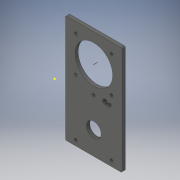
# Autodesk Inventor part: y gearing adapter
Saved by Autodesk Inventor 2019 (Build 230136000, 136)
## iProperties
Created: 2018-07-27
Part Number: y gearing adapter
Material: Generic
Document SubType Name: Modeling
Designer: torba
Density: 1 g/cm^3
Appearance: Gray
Author: torba
Autodesk Inventor part; units mm, degrees
ref_plane "YZ Plane" through (0, 0, 0) normal (1, 0, 0) x (0, 1, 0)
ref_plane "XZ Plane" through (0, 0, 0) normal (0, 1, 0) x (-1, 0, 0)
ref_plane "XY Plane" through (0, 0, 0) normal (0, 0, 1) x (1, 0, 0)
sketch "Sketch1" plane through (0, 0, 0) normal (0, 0, 1) x (1, 0, 0)
  arc A0 (44.2015, -79.5823) -> (38.6015, -79.5823) centre (41.4015, -79.5823) ccw
  arc A1 (38.6015, -85.1823) -> (44.2015, -85.1823) centre (41.4015, -85.1823) ccw
  line L0 (38.6015, -85.1823) -> (38.6015, -79.5823)
  line L1 (44.2015, -79.5823) -> (44.2015, -85.1823)
  arc A2 (39.4335, -50.3778) -> (112.9665, -50.3778) centre (76.2, -50.3778) ccw
  arc A3 (112.9665, -44.7898) -> (39.4335, -44.7898) centre (76.2, -44.7898) ccw
  line L2 (39.4335, -50.3778) -> (39.4335, -44.7898)
  line L3 (112.9665, -44.7898) -> (112.9665, -50.3778)
  line L4 (44.2015, -9.9853) -> (44.2015, -15.5853)
  arc A4 (44.2015, -9.9853) -> (38.6015, -9.9853) centre (41.4015, -9.9853) ccw
  line L5 (38.6015, -15.5853) -> (38.6015, -9.9853)
  arc A5 (38.6015, -15.5853) -> (44.2015, -15.5853) centre (41.4015, -15.5853) ccw
  line L6 (108.1985, -85.1823) -> (108.1985, -79.5823)
  arc A6 (108.1985, -85.1823) -> (113.7985, -85.1823) centre (110.9985, -85.1823) ccw
  line L7 (113.7985, -79.5823) -> (113.7985, -85.1823)
  arc A7 (113.7985, -79.5823) -> (108.1985, -79.5823) centre (110.9985, -79.5823) ccw
  line L8 (108.1985, -15.5853) -> (108.1985, -9.9853)
  arc A8 (113.7985, -9.9853) -> (108.1985, -9.9853) centre (110.9985, -9.9853) ccw
  line L9 (113.7985, -9.9853) -> (113.7985, -15.5853)
  arc A9 (108.1985, -15.5853) -> (113.7985, -15.5853) centre (110.9985, -15.5853) ccw
  circle A10 centre (76.2, -47.5838) radius 1.27
  line L10 (6.35, 0.0014) -> (6.35, -109.7489)
  line L11 (152.4, 0) -> (0, 0)
  line L12 (146.05, 0.0027) -> (146.05, -109.7476)
  line L13 (0, -109.7503) -> (152.4, -109.7503)
  line L14 (21.2, 7.4162) -> (131.2, 7.4162)
  line L15 (131.2, 7.4162) -> (131.2, -102.5838)
  line L16 (131.2, -102.5838) -> (21.2, -102.5838)
  line L17 (21.2, -102.5838) -> (21.2, 7.4162)
  line L18 (21.2, 7.4162) -> (131.2, -102.5838) construction
  line L19 (131.2, 7.4162) -> (21.2, -102.5838) construction
  dimension "d0" = 2.8
  dimension "d1" = 36.7665
  dimension "d2" = 2.54
  dimension "d3" = 90
  dimension "d4" = 90
  dimension "d5" = 90
  dimension "d6" = 90
  dimension "d7" = 109.7503
  dimension "d8" = 32.2515
  dimension "d9" = 33.0835
  dimension "d10" = 101.8485
  dimension "d11" = 139.7
  dimension "d12" = 6.35
  dimension "d13" = 38.6015
  dimension "d14" = 6.35
  dimension "d15" = 0.0027
  dimension "d16" = 37.8515
  dimension "d17" = 109.7476
  dimension "d18" = 9.9853
  dimension "d19" = 69.597
  dimension "d20" = 75.197
  dimension "d21" = 79.5823
  dimension "d22" = 44.7898
  dimension "d23" = 50.3778
  dimension "d24" = 47.5838
  dimension "d25" = 69.85
  dimension "d26" = 9.9853
  dimension "d27" = 79.5823
  dimension "d28" = 0.0014
  dimension "d29" = 109.7489
  dimension "d30" = 146.05
  dimension "d31" = 146.05
  dimension "d32" = 110
  dimension "d33" = 110
  dimension "d34" = 17.4015
  constraints: 40 end point, 24 tangent, 20 point on circle, 11 centre point, 10 parallel, 2 horizontal, 2 midpoint, 1 equal radius, 1 perpendicular, 1 vertical
  measures "d0" radius of A8
  measures "d1" radius of A3
  measures "d2" diameter of A10
  measures "d3" angle of L11 L9
  measures "d4" angle of L11 L8
  measures "d5" angle of L11 L1
  measures "d6" angle of L11 L0
  measures "d7" distance between parallel lines of L11 L13
  measures "d8" distance between parallel lines of L12 L7
  measures "d9" distance between parallel lines of L12 L3
  measures "d10" distance between parallel lines of L12 L4
  measures "d11" distance between parallel lines of L12 L10
  measures "d12" distance from line of L11.start L12
  measures "d13" distance from line of L11.start L9
  measures "d14" distance from line of L13.end L12
  measures "d15" distance from line of L12.start L11
  measures "d16" distance from line of L12.start L8
  measures "d17" distance from line of L12.end L11
  measures "d18" distance from line of L9.start L11
  measures "d19" distance from line of L9.start L1
  measures "d20" distance from line of L9.start L0
  measures "d21" distance from line of L7.start L11
  measures "d22" distance from line of L3.start L11
  measures "d23" distance from line of L3.end L11
  measures "d24" distance from line of A10.centre L11
  measures "d25" distance from line of A10.centre L12
  measures "d26" distance from line of L4.start L11
  measures "d27" distance from line of L1.start L11
  measures "d28" distance from line of L10.start L11
  measures "d29" distance from line of L10.end L11
  measures "d30" distance from line of L11.end L12
  measures "d31" distance from line of L13.start L12
  measures "d32" distance between parallel lines of L15 L17
  measures "d33" distance between parallel lines of L16 L14
  measures "d34" distance from line of L16 A1.centre
extrude "Extrusion1" add sketch "Sketch1" along normal blind 6.35 contours L15 L16 L17 L11 | L11 L17 L14 L15
sketch "Sketch3" plane through (0, 0, 6.35) normal (0, 0, 1) x (1, 0, 0)
  line L0 (112.9665, -44.7898) -> (112.9665, -50.3778) projected
  arc A0 (39.4335, -50.3778) -> (112.9665, -50.3778) centre (76.2, -50.3778) ccw projected
  line L1 (39.4335, -50.3778) -> (39.4335, -44.7898) projected
  arc A1 (112.9665, -44.7898) -> (39.4335, -44.7898) centre (76.2, -44.7898) ccw projected
  arc A2 (38.6015, -15.5853) -> (44.2015, -15.5853) centre (41.4015, -15.5853) ccw projected
  line L2 (38.6015, -15.5853) -> (38.6015, -9.9853) projected
  arc A3 (44.2015, -9.9853) -> (38.6015, -9.9853) centre (41.4015, -9.9853) ccw projected
  line L3 (44.2015, -9.9853) -> (44.2015, -15.5853) projected
  line L4 (44.2015, -79.5823) -> (44.2015, -85.1823) projected
  arc A4 (38.6015, -85.1823) -> (44.2015, -85.1823) centre (41.4015, -85.1823) ccw projected
  line L5 (38.6015, -85.1823) -> (38.6015, -79.5823) projected
  arc A5 (44.2015, -79.5823) -> (38.6015, -79.5823) centre (41.4015, -79.5823) ccw projected
  arc A6 (113.7985, -79.5823) -> (108.1985, -79.5823) centre (110.9985, -79.5823) ccw projected
  line L6 (113.7985, -79.5823) -> (113.7985, -85.1823) projected
  arc A7 (108.1985, -85.1823) -> (113.7985, -85.1823) centre (110.9985, -85.1823) ccw projected
  line L7 (108.1985, -85.1823) -> (108.1985, -79.5823) projected
  arc A8 (113.7985, -9.9853) -> (108.1985, -9.9853) centre (110.9985, -9.9853) ccw projected
  line L8 (113.7985, -9.9853) -> (113.7985, -15.5853) projected
  arc A9 (108.1985, -15.5853) -> (113.7985, -15.5853) centre (110.9985, -15.5853) ccw projected
  line L9 (108.1985, -15.5853) -> (108.1985, -9.9853) projected
  line L10 (131.2, 7.4162) -> (21.2, 7.4162) projected
  line L11 (21.2, 7.4162) -> (21.2, -102.5838) projected
  line L12 (21.2, -102.5838) -> (131.2, -102.5838) projected
  line L13 (131.2, -102.5838) -> (131.2, 7.4162) projected
  line L14 (112.9665, 65.2102) -> (112.9665, 59.6222)
  arc A10 (39.4335, 59.6222) -> (112.9665, 59.6222) centre (76.2, 59.6222) ccw
  line L15 (39.4335, 59.6222) -> (39.4335, 65.2102)
  arc A11 (112.9665, 65.2102) -> (39.4335, 65.2102) centre (76.2, 65.2102) ccw
  arc A12 (38.6015, 94.4147) -> (44.2015, 94.4147) centre (41.4015, 94.4147) ccw
  line L16 (38.6015, 94.4147) -> (38.6015, 100.0147)
  arc A13 (44.2015, 100.0147) -> (38.6015, 100.0147) centre (41.4015, 100.0147) ccw
  line L17 (44.2015, 100.0147) -> (44.2015, 94.4147)
  line L18 (44.2015, 30.4177) -> (44.2015, 24.8177)
  arc A14 (38.6015, 24.8177) -> (44.2015, 24.8177) centre (41.4015, 24.8177) ccw
  line L19 (38.6015, 24.8177) -> (38.6015, 30.4177)
  arc A15 (44.2015, 30.4177) -> (38.6015, 30.4177) centre (41.4015, 30.4177) ccw
  arc A16 (113.7985, 30.4177) -> (108.1985, 30.4177) centre (110.9985, 30.4177) ccw
  line L20 (113.7985, 30.4177) -> (113.7985, 24.8177)
  arc A17 (108.1985, 24.8177) -> (113.7985, 24.8177) centre (110.9985, 24.8177) ccw
  line L21 (108.1985, 24.8177) -> (108.1985, 30.4177)
  arc A18 (113.7985, 100.0147) -> (108.1985, 100.0147) centre (110.9985, 100.0147) ccw
  line L22 (113.7985, 100.0147) -> (113.7985, 94.4147)
  arc A19 (108.1985, 94.4147) -> (113.7985, 94.4147) centre (110.9985, 94.4147) ccw
  line L23 (108.1985, 94.4147) -> (108.1985, 100.0147)
  line L24 (131.2, 117.4162) -> (21.2, 117.4162)
  line L25 (21.2, 117.4162) -> (21.2, 7.4162)
  line L26 (21.2, 7.4162) -> (131.2, 7.4162)
  line L27 (131.2, 7.4162) -> (131.2, 117.4162)
  point P0 (0, 0)
  dimension "d37" = 90
  dimension "d38" = 90
  dimension "d39" = 90
  dimension "d40" = 90
  dimension "d41" = 90
  dimension "d42" = 90
  dimension "d43" = 90
  dimension "d44" = 90
  dimension "d45" = 90
  dimension "d46" = 90
  dimension "d47" = 90
  dimension "d48" = 90
  dimension "d49" = 90
  dimension "d50" = 110
  dimension "d51" = 0
  dimension "d52" = 17.4015
  dimension "d53" = 17.4015
  dimension "d54" = 18.2335
  dimension "d55" = 23.0015
  dimension "d56" = 23.0015
  dimension "d57" = 86.9985
  dimension "d58" = 86.9985
  dimension "d59" = 91.7665
  dimension "d60" = 92.5985
  dimension "d61" = 92.5985
  dimension "d62" = 110
  dimension "d63" = 0
  dimension "d64" = 92.5985
  dimension "d65" = 23.0015
  dimension "d66" = 57.794
  dimension "d67" = 52.206
  dimension "d68" = 92.5985
  dimension "d69" = 23.0015
  constraints: 28 end point, 24 tangent, 20 point on circle, 10 centre point, 1 parallel
  measures "d37" angle of L10 L27
  measures "d38" angle of L10 L22
  measures "d39" angle of L10 L20
  measures "d40" angle of L10 L14
  measures "d41" angle of L10 L23
  measures "d42" angle of L10 L21
  measures "d43" angle of L10 L17
  measures "d44" angle of L10 L18
  measures "d45" angle of L10 L15
  measures "d46" angle of L10 L16
  measures "d47" angle of L10 L19
  measures "d48" angle of L10 L25
  measures "d49" angle of L13 L26
  measures "d50" distance between parallel lines of L10 L24
  measures "d51" distance from line of L10.start L27
  measures "d52" distance from line of L10.start L22
  measures "d53" distance from line of L10.start L20
  measures "d54" distance from line of L10.start L14
  measures "d55" distance from line of L10.start L23
  measures "d56" distance from line of L10.start L21
  measures "d57" distance from line of L10.start L17
  measures "d58" distance from line of L10.start L18
  measures "d59" distance from line of L10.start L15
  measures "d60" distance from line of L10.start L16
  measures "d61" distance from line of L10.start L19
  measures "d62" distance from line of L10.start L25
  measures "d63" distance from line of L10.start L26
  measures "d64" distance from line of L22.start L10
  measures "d65" distance from line of L20.start L10
  measures "d66" distance from line of L14.start L10
  measures "d67" distance from line of L14.end L10
  measures "d68" distance from line of L17.start L10
  measures "d69" distance from line of L18.start L10
extrude "Extrusion2" add sketch "Sketch3" against normal blind 6.35 contours L10 L25 L24 L27
sketch "Sketch4" plane through (0, 0, 6.35) normal (0, 0, 1) x (1, 0, 0)
  arc A0 (44.2015, 30.4177) -> (38.6015, 30.4177) centre (41.4015, 30.4177) ccw projected
  line L0 (44.2015, 30.4177) -> (44.2015, 24.8177) projected
  arc A1 (38.6015, 24.8177) -> (44.2015, 24.8177) centre (41.4015, 24.8177) ccw projected
  line L1 (38.6015, 24.8177) -> (38.6015, 30.4177) projected
  line L2 (113.7985, 100.0147) -> (113.7985, 94.4147) projected
  arc A2 (108.1985, 94.4147) -> (113.7985, 94.4147) centre (110.9985, 94.4147) ccw projected
  line L3 (108.1985, 94.4147) -> (108.1985, 100.0147) projected
  arc A3 (113.7985, 100.0147) -> (108.1985, 100.0147) centre (110.9985, 100.0147) ccw projected
  line L4 (44.2015, 100.0147) -> (44.2015, 94.4147) projected
  arc A4 (38.6015, 94.4147) -> (44.2015, 94.4147) centre (41.4015, 94.4147) ccw projected
  line L5 (38.6015, 94.4147) -> (38.6015, 100.0147) projected
  arc A5 (44.2015, 100.0147) -> (38.6015, 100.0147) centre (41.4015, 100.0147) ccw projected
  line L6 (108.1985, 24.8177) -> (108.1985, 30.4177) projected
  arc A6 (113.7985, 30.4177) -> (108.1985, 30.4177) centre (110.9985, 30.4177) ccw projected
  line L7 (113.7985, 30.4177) -> (113.7985, 24.8177) projected
  arc A7 (108.1985, 24.8177) -> (113.7985, 24.8177) centre (110.9985, 24.8177) ccw projected
  arc A8 (112.9665, 65.2102) -> (39.4335, 65.2102) centre (76.2, 65.2102) ccw projected
  line L8 (112.9665, 65.2102) -> (112.9665, 59.6222) projected
  arc A9 (39.4335, 59.6222) -> (112.9665, 59.6222) centre (76.2, 59.6222) ccw projected
  line L9 (39.4335, 59.6222) -> (39.4335, 65.2102) projected
  line L10 (112.9665, -44.7898) -> (112.9665, -50.3778) projected
  arc A10 (39.4335, -50.3778) -> (112.9665, -50.3778) centre (76.2, -50.3778) ccw projected
  line L11 (39.4335, -50.3778) -> (39.4335, -44.7898) projected
  arc A11 (112.9665, -44.7898) -> (39.4335, -44.7898) centre (76.2, -44.7898) ccw projected
  arc A12 (38.6015, -15.5853) -> (44.2015, -15.5853) centre (41.4015, -15.5853) ccw projected
  line L12 (38.6015, -15.5853) -> (38.6015, -9.9853) projected
  arc A13 (44.2015, -9.9853) -> (38.6015, -9.9853) centre (41.4015, -9.9853) ccw projected
  line L13 (44.2015, -9.9853) -> (44.2015, -15.5853) projected
  line L14 (44.2015, -79.5823) -> (44.2015, -85.1823) projected
  arc A14 (38.6015, -85.1823) -> (44.2015, -85.1823) centre (41.4015, -85.1823) ccw projected
  line L15 (38.6015, -85.1823) -> (38.6015, -79.5823) projected
  arc A15 (44.2015, -79.5823) -> (38.6015, -79.5823) centre (41.4015, -79.5823) ccw projected
  arc A16 (113.7985, -79.5823) -> (108.1985, -79.5823) centre (110.9985, -79.5823) ccw projected
  line L16 (113.7985, -79.5823) -> (113.7985, -85.1823) projected
  arc A17 (108.1985, -85.1823) -> (113.7985, -85.1823) centre (110.9985, -85.1823) ccw projected
  line L17 (108.1985, -85.1823) -> (108.1985, -79.5823) projected
  arc A18 (113.7985, -9.9853) -> (108.1985, -9.9853) centre (110.9985, -9.9853) ccw projected
  line L18 (113.7985, -9.9853) -> (113.7985, -15.5853) projected
  arc A19 (108.1985, -15.5853) -> (113.7985, -15.5853) centre (110.9985, -15.5853) ccw projected
  line L19 (108.1985, -15.5853) -> (108.1985, -9.9853) projected
  line L20 (21.2, -102.5838) -> (21.2, 117.4162) projected
  line L21 (21.2, -102.5838) -> (131.2, -102.5838) projected
  line L22 (131.2, -102.5838) -> (131.2, 117.4162) projected
  line L23 (21.2, 117.4162) -> (131.2, 117.4162) projected
  line L24 (76.2, -50.3778) -> (76.2, -44.7898)
  line L25 (76.2, 59.6222) -> (76.2, 65.2102)
  circle A20 centre (76.2, -47.5838) radius 0.5
  circle A21 centre (76.2, 62.4162) radius 0.5
  point P0 (0, 0)
  dimension "d72" = 1
  dimension "d73" = 1
  constraints: 4 end point, 2 centre point, 2 midpoint, 2 vertical
  measures "d72" diameter of A20
  measures "d73" diameter of A21
extrude "Extrusion3" add sketch "Sketch4" against normal blind 6.35 contours A20 L24 | L24 A20 | A21 L25 | L25 A21
sketch "Sketch6" plane through (21.2, -102.5838, 0) normal (0, -1, 0) x (1, 0, 0)
  line L0 (110, 0) -> (0, 0) projected
  line L1 (110, 0) -> (0, 0) projected
  line L2 (110, 0) -> (110, 6.35) projected
  line L3 (0, 6.35) -> (110, 6.35) projected
  line L4 (0, 0) -> (0, 6.35) projected
  point P0 (-21.2, 0)
extrude "Extrusion4" cut sketch "Sketch6" against normal blind 10
sketch "Sketch7" plane through (0, 0, 6.35) normal (0, 0, 1) x (1, 0, 0)
  line L0 (21.2, -92.5838) -> (131.2, -92.5838) projected
  line L1 (131.2, -92.5838) -> (131.2, 117.4162) projected
  line L2 (21.2, 117.4162) -> (131.2, 117.4162) projected
  line L3 (21.2, -92.5838) -> (21.2, 117.4162) projected
  arc A0 (113.7985, -9.9853) -> (108.1985, -9.9853) centre (110.9985, -9.9853) ccw projected
  line L4 (113.7985, -9.9853) -> (113.7985, -15.5853) projected
  arc A1 (108.1985, -15.5853) -> (113.7985, -15.5853) centre (110.9985, -15.5853) ccw projected
  line L5 (108.1985, -15.5853) -> (108.1985, -9.9853) projected
  arc A2 (113.7985, -79.5823) -> (108.1985, -79.5823) centre (110.9985, -79.5823) ccw projected
  line L6 (113.7985, -79.5823) -> (113.7985, -85.1823) projected
  arc A3 (108.1985, -85.1823) -> (113.7985, -85.1823) centre (110.9985, -85.1823) ccw projected
  line L7 (108.1985, -85.1823) -> (108.1985, -79.5823) projected
  line L8 (44.2015, -79.5823) -> (44.2015, -85.1823) projected
  arc A4 (38.6015, -85.1823) -> (44.2015, -85.1823) centre (41.4015, -85.1823) ccw projected
  line L9 (38.6015, -85.1823) -> (38.6015, -79.5823) projected
  arc A5 (44.2015, -79.5823) -> (38.6015, -79.5823) centre (41.4015, -79.5823) ccw projected
  arc A6 (38.6015, -15.5853) -> (44.2015, -15.5853) centre (41.4015, -15.5853) ccw projected
  line L10 (38.6015, -15.5853) -> (38.6015, -9.9853) projected
  arc A7 (44.2015, -9.9853) -> (38.6015, -9.9853) centre (41.4015, -9.9853) ccw projected
  line L11 (44.2015, -9.9853) -> (44.2015, -15.5853) projected
  line L12 (112.9665, -44.7898) -> (112.9665, -50.3778) projected
  arc A8 (39.4335, -50.3778) -> (112.9665, -50.3778) centre (76.2, -50.3778) ccw projected
  line L13 (39.4335, -50.3778) -> (39.4335, -44.7898) projected
  arc A9 (112.9665, -44.7898) -> (39.4335, -44.7898) centre (76.2, -44.7898) ccw projected
  arc A10 (112.9665, 65.2102) -> (39.4335, 65.2102) centre (76.2, 65.2102) ccw projected
  line L14 (112.9665, 65.2102) -> (112.9665, 59.6222) projected
  arc A11 (39.4335, 59.6222) -> (112.9665, 59.6222) centre (76.2, 59.6222) ccw projected
  line L15 (39.4335, 59.6222) -> (39.4335, 65.2102) projected
  line L16 (108.1985, 24.8177) -> (108.1985, 30.4177) projected
  arc A12 (113.7985, 30.4177) -> (108.1985, 30.4177) centre (110.9985, 30.4177) ccw projected
  line L17 (113.7985, 30.4177) -> (113.7985, 24.8177) projected
  arc A13 (108.1985, 24.8177) -> (113.7985, 24.8177) centre (110.9985, 24.8177) ccw projected
  line L18 (44.2015, 100.0147) -> (44.2015, 94.4147) projected
  arc A14 (38.6015, 94.4147) -> (44.2015, 94.4147) centre (41.4015, 94.4147) ccw projected
  line L19 (38.6015, 94.4147) -> (38.6015, 100.0147) projected
  arc A15 (44.2015, 100.0147) -> (38.6015, 100.0147) centre (41.4015, 100.0147) ccw projected
  line L20 (113.7985, 100.0147) -> (113.7985, 94.4147) projected
  arc A16 (108.1985, 94.4147) -> (113.7985, 94.4147) centre (110.9985, 94.4147) ccw projected
  line L21 (108.1985, 94.4147) -> (108.1985, 100.0147) projected
  arc A17 (113.7985, 100.0147) -> (108.1985, 100.0147) centre (110.9985, 100.0147) ccw projected
  arc A18 (44.2015, 30.4177) -> (38.6015, 30.4177) centre (41.4015, 30.4177) ccw projected
  line L22 (44.2015, 30.4177) -> (44.2015, 24.8177) projected
  arc A19 (38.6015, 24.8177) -> (44.2015, 24.8177) centre (41.4015, 24.8177) ccw projected
  line L23 (38.6015, 24.8177) -> (38.6015, 30.4177) projected
  point P0 (0, 0)
extrude "Extrusion5" add sketch "Sketch7" against normal up to surface (6.35 mm away) contours L12 A8 L13 A9
sketch "Sketch8" plane through (0, 0, 6.35) normal (0, 0, 1) x (1, 0, 0)
  point P0 (0, 0)
hole "Hole1" at (76.2, -47.5838, 6.35) direction (0, 0, -1) diameter 28.575 end through all
sketch "Sketch9" plane through (0, 0, 6.35) normal (0, 0, 1) x (1, 0, 0)
  circle A0 centre (76.2, -47.5838) radius 14.2875 construction
  arc A1 (44.2015, 30.4177) -> (38.6015, 30.4177) centre (41.4015, 30.4177) ccw projected
  line L0 (44.2015, 30.4177) -> (44.2015, 24.8177) projected
  arc A2 (38.6015, 24.8177) -> (44.2015, 24.8177) centre (41.4015, 24.8177) ccw projected
  line L1 (38.6015, 24.8177) -> (38.6015, 30.4177) projected
  line L2 (113.7985, 100.0147) -> (113.7985, 94.4147) projected
  arc A3 (108.1985, 94.4147) -> (113.7985, 94.4147) centre (110.9985, 94.4147) ccw projected
  line L3 (108.1985, 94.4147) -> (108.1985, 100.0147) projected
  arc A4 (113.7985, 100.0147) -> (108.1985, 100.0147) centre (110.9985, 100.0147) ccw projected
  line L4 (44.2015, 100.0147) -> (44.2015, 94.4147) projected
  arc A5 (38.6015, 94.4147) -> (44.2015, 94.4147) centre (41.4015, 94.4147) ccw projected
  line L5 (38.6015, 94.4147) -> (38.6015, 100.0147) projected
  arc A6 (44.2015, 100.0147) -> (38.6015, 100.0147) centre (41.4015, 100.0147) ccw projected
  line L6 (108.1985, 24.8177) -> (108.1985, 30.4177) projected
  arc A7 (113.7985, 30.4177) -> (108.1985, 30.4177) centre (110.9985, 30.4177) ccw projected
  line L7 (113.7985, 30.4177) -> (113.7985, 24.8177) projected
  arc A8 (108.1985, 24.8177) -> (113.7985, 24.8177) centre (110.9985, 24.8177) ccw projected
  arc A9 (112.9665, 65.2102) -> (39.4335, 65.2102) centre (76.2, 65.2102) ccw projected
  line L8 (112.9665, 65.2102) -> (112.9665, 59.6222) projected
  arc A10 (39.4335, 59.6222) -> (112.9665, 59.6222) centre (76.2, 59.6222) ccw projected
  line L9 (39.4335, 59.6222) -> (39.4335, 65.2102) projected
  arc A11 (38.6015, -15.5853) -> (44.2015, -15.5853) centre (41.4015, -15.5853) ccw construction
  line L10 (38.6015, -15.5853) -> (38.6015, -9.9853) construction
  arc A12 (44.2015, -9.9853) -> (38.6015, -9.9853) centre (41.4015, -9.9853) ccw construction
  line L11 (44.2015, -9.9853) -> (44.2015, -15.5853) construction
  line L12 (44.2015, -79.5823) -> (44.2015, -85.1823) construction
  arc A13 (38.6015, -85.1823) -> (44.2015, -85.1823) centre (41.4015, -85.1823) ccw construction
  line L13 (38.6015, -85.1823) -> (38.6015, -79.5823) construction
  arc A14 (44.2015, -79.5823) -> (38.6015, -79.5823) centre (41.4015, -79.5823) ccw construction
  arc A15 (113.7985, -79.5823) -> (108.1985, -79.5823) centre (110.9985, -79.5823) ccw construction
  line L14 (113.7985, -79.5823) -> (113.7985, -85.1823) construction
  arc A16 (108.1985, -85.1823) -> (113.7985, -85.1823) centre (110.9985, -85.1823) ccw construction
  line L15 (108.1985, -85.1823) -> (108.1985, -79.5823) construction
  arc A17 (113.7985, -9.9853) -> (108.1985, -9.9853) centre (110.9985, -9.9853) ccw construction
  line L16 (113.7985, -9.9853) -> (113.7985, -15.5853) construction
  arc A18 (108.1985, -15.5853) -> (113.7985, -15.5853) centre (110.9985, -15.5853) ccw construction
  line L17 (108.1985, -15.5853) -> (108.1985, -9.9853) construction
  line L18 (21.2, -92.5838) -> (131.2, -92.5838) projected
  line L19 (131.2, -92.5838) -> (131.2, 117.4162) projected
  line L20 (21.2, 117.4162) -> (131.2, 117.4162) projected
  line L21 (21.2, -92.5838) -> (21.2, 117.4162) projected
  line L22 (41.4015, -85.1823) -> (41.4015, -79.5823) construction
  line L23 (41.4015, -15.5853) -> (41.4015, -9.9853) construction
  line L24 (110.9985, -85.1823) -> (110.9985, -79.5823) construction
  line L25 (110.9985, -15.5853) -> (110.9985, -9.9853) construction
  circle A19 centre (41.4015, -82.3823) radius 2.8
  circle A20 centre (41.4015, -12.7853) radius 2.8
  circle A21 centre (110.9985, -12.7853) radius 2.8
  line L26 (108.1985, -9.9853) -> (108.1985, -15.5853) projected
  circle A22 centre (110.9985, -82.3823) radius 2.8
  line L27 (41.4015, -85.1823) -> (41.4015, -79.5823) construction
  line L28 (44.2015, -85.1823) -> (44.2015, -79.5823)
  line L29 (38.6015, -79.5823) -> (38.6015, -85.1823)
  arc A23 (38.6015, -85.1823) -> (44.2015, -85.1823) centre (41.4015, -85.1823) ccw
  arc A24 (44.2015, -79.5823) -> (38.6015, -79.5823) centre (41.4015, -79.5823) ccw
  line L30 (41.4015, -15.5853) -> (41.4015, -9.9853) construction
  line L31 (44.2015, -15.5853) -> (44.2015, -9.9853)
  line L32 (38.6015, -9.9853) -> (38.6015, -15.5853)
  arc A25 (38.6015, -15.5853) -> (44.2015, -15.5853) centre (41.4015, -15.5853) ccw
  arc A26 (44.2015, -9.9853) -> (38.6015, -9.9853) centre (41.4015, -9.9853) ccw
  line L33 (110.9985, -85.1823) -> (110.9985, -79.5823) construction
  line L34 (113.7985, -85.1823) -> (113.7985, -79.5823)
  line L35 (108.1985, -79.5823) -> (108.1985, -85.1823)
  arc A27 (108.1985, -85.1823) -> (113.7985, -85.1823) centre (110.9985, -85.1823) ccw
  arc A28 (113.7985, -79.5823) -> (108.1985, -79.5823) centre (110.9985, -79.5823) ccw
  line L36 (110.9985, -15.5853) -> (110.9985, -9.9853) construction
  line L37 (113.7985, -15.5853) -> (113.7985, -9.9853)
  line L38 (108.1985, -9.9853) -> (108.1985, -15.5853)
  arc A29 (108.1985, -15.5853) -> (113.7985, -15.5853) centre (110.9985, -15.5853) ccw
  arc A30 (113.7985, -9.9853) -> (108.1985, -9.9853) centre (110.9985, -9.9853) ccw
  point P0 (0, 0)
  point P1 (41.4015, -12.7853)
  constraints: 40 end point, 20 tangent, 16 point on circle, 12 centre point, 8 equal length, 8 midpoint, 4 vertical, 1 concentric
extrude "Extrusion6" add sketch "Sketch9" against normal blind 6.35 contours L28 A23 L29 A19 | A19 L29 A24 L28 | L31 A25 L32 A20 | A20 L32 A26 L31 | L37 A29 L26 A21 | A21 L26 A30 L37 | L34 A27 L35 A22 | A22 L35 A28 L34
sketch "Sketch10" plane through (0, 0, 6.35) normal (0, 0, 1) x (1, 0, 0)
  circle A0 centre (110.9985, -82.3823) radius 2.8 projected
  circle A1 centre (110.9985, -12.7853) radius 2.8 projected
  circle A2 centre (76.2, -47.5838) radius 14.2875 projected
  arc A3 (44.2015, 30.4177) -> (38.6015, 30.4177) centre (41.4015, 30.4177) ccw projected
  line L0 (44.2015, 30.4177) -> (44.2015, 24.8177) projected
  arc A4 (38.6015, 24.8177) -> (44.2015, 24.8177) centre (41.4015, 24.8177) ccw projected
  line L1 (38.6015, 24.8177) -> (38.6015, 30.4177) projected
  line L2 (113.7985, 100.0147) -> (113.7985, 94.4147) projected
  arc A5 (108.1985, 94.4147) -> (113.7985, 94.4147) centre (110.9985, 94.4147) ccw projected
  line L3 (108.1985, 94.4147) -> (108.1985, 100.0147) projected
  arc A6 (113.7985, 100.0147) -> (108.1985, 100.0147) centre (110.9985, 100.0147) ccw projected
  line L4 (44.2015, 100.0147) -> (44.2015, 94.4147) projected
  arc A7 (38.6015, 94.4147) -> (44.2015, 94.4147) centre (41.4015, 94.4147) ccw projected
  line L5 (38.6015, 94.4147) -> (38.6015, 100.0147) projected
  arc A8 (44.2015, 100.0147) -> (38.6015, 100.0147) centre (41.4015, 100.0147) ccw projected
  line L6 (108.1985, 24.8177) -> (108.1985, 30.4177) projected
  arc A9 (113.7985, 30.4177) -> (108.1985, 30.4177) centre (110.9985, 30.4177) ccw projected
  line L7 (113.7985, 30.4177) -> (113.7985, 24.8177) projected
  arc A10 (108.1985, 24.8177) -> (113.7985, 24.8177) centre (110.9985, 24.8177) ccw projected
  arc A11 (112.9665, 65.2102) -> (39.4335, 65.2102) centre (76.2, 65.2102) ccw projected
  line L8 (112.9665, 65.2102) -> (112.9665, 59.6222) projected
  arc A12 (39.4335, 59.6222) -> (112.9665, 59.6222) centre (76.2, 59.6222) ccw projected
  line L9 (39.4335, 59.6222) -> (39.4335, 65.2102) projected
  circle A13 centre (41.4015, -12.7853) radius 2.8 projected
  circle A14 centre (41.4015, -82.3823) radius 2.8 projected
  line L10 (21.2, -92.5838) -> (131.2, -92.5838) projected
  line L11 (131.2, -92.5838) -> (131.2, 117.4162) projected
  line L12 (21.2, 117.4162) -> (131.2, 117.4162) projected
  line L13 (21.2, -92.5838) -> (21.2, 117.4162) projected
  point P0 (0, 0)
sketch "Sketch11" plane through (0, 0, 6.35) normal (0, 0, 1) x (1, 0, 0)
  circle A0 centre (76.2, 62.4162) radius 16
  circle A1 centre (76.2, -47.5838) radius 43.0506
  circle A2 centre (110.9985, -82.3823) radius 2.8 projected
  circle A3 centre (110.9985, -12.7853) radius 2.8 projected
  circle A4 centre (76.2, -47.5838) radius 14.2875 projected
  arc A5 (44.2015, 30.4177) -> (38.6015, 30.4177) centre (41.4015, 30.4177) ccw construction
  line L0 (44.2015, 30.4177) -> (44.2015, 24.8177) construction
  arc A6 (38.6015, 24.8177) -> (44.2015, 24.8177) centre (41.4015, 24.8177) ccw construction
  line L1 (38.6015, 24.8177) -> (38.6015, 30.4177) construction
  line L2 (113.7985, 100.0147) -> (113.7985, 94.4147) construction
  arc A7 (108.1985, 94.4147) -> (113.7985, 94.4147) centre (110.9985, 94.4147) ccw construction
  line L3 (108.1985, 94.4147) -> (108.1985, 100.0147) construction
  arc A8 (113.7985, 100.0147) -> (108.1985, 100.0147) centre (110.9985, 100.0147) ccw construction
  line L4 (44.2015, 100.0147) -> (44.2015, 94.4147) construction
  arc A9 (38.6015, 94.4147) -> (44.2015, 94.4147) centre (41.4015, 94.4147) ccw construction
  line L5 (38.6015, 94.4147) -> (38.6015, 100.0147) construction
  arc A10 (44.2015, 100.0147) -> (38.6015, 100.0147) centre (41.4015, 100.0147) ccw construction
  line L6 (108.1985, 24.8177) -> (108.1985, 30.4177) construction
  arc A11 (113.7985, 30.4177) -> (108.1985, 30.4177) centre (110.9985, 30.4177) ccw construction
  line L7 (113.7985, 30.4177) -> (113.7985, 24.8177) construction
  arc A12 (108.1985, 24.8177) -> (113.7985, 24.8177) centre (110.9985, 24.8177) ccw construction
  arc A13 (112.9665, 65.2102) -> (39.4335, 65.2102) centre (76.2, 65.2102) ccw construction
  line L8 (112.9665, 65.2102) -> (112.9665, 59.6222) construction
  arc A14 (39.4335, 59.6222) -> (112.9665, 59.6222) centre (76.2, 59.6222) ccw construction
  line L9 (39.4335, 59.6222) -> (39.4335, 65.2102) construction
  circle A15 centre (41.4015, -12.7853) radius 2.8 projected
  circle A16 centre (41.4015, -82.3823) radius 2.8 projected
  line L10 (21.2, -92.5838) -> (131.2, -92.5838) projected
  line L11 (131.2, -92.5838) -> (131.2, 117.4162) projected
  line L12 (21.2, 117.4162) -> (131.2, 117.4162) construction
  line L13 (21.2, -92.5838) -> (21.2, 117.4162) projected
  circle A17 centre (76.2, 62.4162) radius 0.5 construction
  line L14 (112.9665, 59.6222) -> (112.9665, 65.2102) construction
  line L15 (110.9985, 94.4147) -> (110.9985, 100.0147) construction
  line L16 (110.9985, 33.2177) -> (110.9985, 91.6147) construction
  line L17 (110.9985, 24.8177) -> (110.9985, 30.4177) construction
  line L18 (110.9985, 33.2177) -> (110.9985, 77.0778) construction
  circle A18 centre (110.9985, 97.2147) radius 2.8
  circle A19 centre (110.9985, 27.6177) radius 2.8
  circle A20 centre (41.4015, 27.6177) radius 2.8
  circle A21 centre (41.4015, 97.2147) radius 2.8
  line L19 (41.4015, 94.4147) -> (41.4015, 91.6147) construction
  line L20 (41.4015, 33.2177) -> (41.4015, 30.4177) construction
  line L21 (41.4015, 100.0147) -> (41.4015, 91.6147) construction
  line L22 (41.4015, 33.2177) -> (41.4015, 24.8177) construction
  point P0 (0, 0)
  dimension "d91" = 32
  dimension "d92" = 86.1011
  dimension "d93" = 20.2015
  dimension "d95" = 86.9985
  dimension "d96" = 17.4015
  dimension "d97" = 23.0015
  dimension "d99" = 20.2015
  dimension "d100" = 89.7985
  dimension "d101" = 20.2015
  dimension "d102" = 89.7985
  constraints: 17 end point, 8 parallel, 7 tangent, 6 centre point, 5 point on circle, 2 concentric, 2 midpoint, 1 point on line
  measures "d91" diameter of A0
  measures "d92" diameter of A1
  measures "d93" distance between parallel lines of L11 L18
  measures "d95" distance from line of L17.end L12
  measures "d96" distance from line of L21.start L12
  measures "d97" distance from line of L19.start L12
  measures "d99" distance from line of A18.centre L12
  measures "d100" distance from line of A19.centre L12
  measures "d101" distance from line of A21.centre L12
  measures "d102" distance from line of A20.centre L12
sketch "Sketch12" plane through (0, 0, 6.35) normal (0, 0, 1) x (1, 0, 0)
  circle A0 centre (110.9985, -82.3823) radius 2.8 projected
  circle A1 centre (110.9985, -12.7853) radius 2.8 projected
  circle A2 centre (76.2, -47.5838) radius 14.2875 projected
  arc A3 (44.2015, 30.4177) -> (38.6015, 30.4177) centre (41.4015, 30.4177) ccw projected
  line L0 (44.2015, 30.4177) -> (44.2015, 24.8177) projected
  arc A4 (38.6015, 24.8177) -> (44.2015, 24.8177) centre (41.4015, 24.8177) ccw projected
  line L1 (38.6015, 24.8177) -> (38.6015, 30.4177) projected
  line L2 (113.7985, 100.0147) -> (113.7985, 94.4147) projected
  arc A5 (108.1985, 94.4147) -> (113.7985, 94.4147) centre (110.9985, 94.4147) ccw projected
  line L3 (108.1985, 94.4147) -> (108.1985, 100.0147) projected
  arc A6 (113.7985, 100.0147) -> (108.1985, 100.0147) centre (110.9985, 100.0147) ccw projected
  line L4 (44.2015, 100.0147) -> (44.2015, 94.4147) projected
  arc A7 (38.6015, 94.4147) -> (44.2015, 94.4147) centre (41.4015, 94.4147) ccw projected
  line L5 (38.6015, 94.4147) -> (38.6015, 100.0147) projected
  arc A8 (44.2015, 100.0147) -> (38.6015, 100.0147) centre (41.4015, 100.0147) ccw projected
  line L6 (108.1985, 24.8177) -> (108.1985, 30.4177) projected
  arc A9 (113.7985, 30.4177) -> (108.1985, 30.4177) centre (110.9985, 30.4177) ccw projected
  line L7 (113.7985, 30.4177) -> (113.7985, 24.8177) projected
  arc A10 (108.1985, 24.8177) -> (113.7985, 24.8177) centre (110.9985, 24.8177) ccw projected
  arc A11 (112.9665, 65.2102) -> (39.4335, 65.2102) centre (76.2, 65.2102) ccw projected
  line L8 (112.9665, 65.2102) -> (112.9665, 59.6222) projected
  arc A12 (39.4335, 59.6222) -> (112.9665, 59.6222) centre (76.2, 59.6222) ccw projected
  line L9 (39.4335, 59.6222) -> (39.4335, 65.2102) projected
  circle A13 centre (41.4015, -12.7853) radius 2.8 projected
  circle A14 centre (41.4015, -82.3823) radius 2.8 projected
  line L10 (21.2, -92.5838) -> (131.2, -92.5838) projected
  line L11 (131.2, -92.5838) -> (131.2, 117.4162) projected
  line L12 (21.2, 117.4162) -> (131.2, 117.4162) projected
  line L13 (21.2, -92.5838) -> (21.2, 117.4162) projected
  line L14 (110.9985, 100.0147) -> (110.9985, 94.4147)
  arc A15 (113.7985, 30.4177) -> (108.1985, 30.4177) centre (110.9985, 30.4177) ccw projected
  line L15 (110.9985, 30.4177) -> (110.9985, 24.8177)
  line L16 (41.4015, 100.0147) -> (41.4015, 94.4147)
  line L17 (41.4015, 30.4177) -> (41.4015, 24.8177)
  circle A16 centre (110.9985, 97.2147) radius 2.8
  circle A17 centre (110.9985, 27.6177) radius 2.8
  line L18 (113.7985, 24.8177) -> (113.7985, 30.4177) projected
  circle A18 centre (41.4015, 27.6177) radius 2.8
  circle A19 centre (41.4015, 97.2147) radius 2.8
  circle A20 centre (76.2, 62.4162) radius 0.5 projected
  circle A21 centre (76.2, 62.4162) radius 36.7665
  line L19 (112.9665, 59.6222) -> (112.9665, 65.2102) projected
  point P0 (0, 0)
  dimension "d103" = 89.7985
  constraints: 8 end point, 6 tangent, 5 centre point, 4 vertical, 3 midpoint, 1 coincident
  measures "d103" distance from line of A17.centre L12
extrude "Extrusion7" add sketch "Sketch12" against normal blind 6.35 contours L0 A18 L1 A3 | L0 A4 L1 A18 | L2 A16 L3 A6 | L2 A5 L3 A16 | L4 A19 L5 A8 | L4 A7 L5 A19 | L6 A17 L7 A10 | L6 A9 L7 A17 | L8 A21 L9 A11 | L8 A12 L9 A21
sketch "Sketch13" plane through (0, 0, 6.35) normal (0, 0, 1) x (1, 0, 0)
  circle A0 centre (76.2, 62.4162) radius 16
  circle A1 centre (76.2, -47.5838) radius 43.0506
  circle A2 centre (76.2, 62.4162) radius 36.7665 projected
  circle A3 centre (41.4015, 27.6177) radius 2.8 projected
  circle A4 centre (110.9985, -82.3823) radius 2.8 projected
  circle A5 centre (110.9985, -12.7853) radius 2.8 projected
  circle A6 centre (76.2, -47.5838) radius 14.2875 projected
  circle A7 centre (110.9985, 97.2147) radius 2.8 projected
  circle A8 centre (41.4015, 97.2147) radius 2.8 projected
  circle A9 centre (110.9985, 27.6177) radius 2.8 projected
  circle A10 centre (76.2, 62.4162) radius 36.7665 projected
  circle A11 centre (41.4015, -12.7853) radius 2.8 projected
  circle A12 centre (41.4015, -82.3823) radius 2.8 projected
  line L0 (21.2, -92.5838) -> (131.2, -92.5838) projected
  line L1 (131.2, -92.5838) -> (131.2, 117.4162) projected
  line L2 (21.2, 117.4162) -> (131.2, 117.4162) projected
  line L3 (21.2, -92.5838) -> (21.2, 117.4162) projected
  line L4 (91.7087, 66.3508) -> (117.9285, -36.9971) construction
  line L5 (60.6913, 66.3508) -> (34.4715, -36.9971)
  circle A13 centre (76.2, 62.4162) radius 36.7665 projected
  line L6 (76.2, 25.6497) -> (76.2, -4.5332) construction
  circle A14 centre (76.2, 10.5582) radius 2.8
  circle A15 centre (76.2, 62.4162) radius 0.5 projected
  circle A16 centre (76.2, 62.4162) radius 12.68
  circle A17 centre (76.2, -47.5838) radius 40.27
  line L7 (76.2, 10.5582) -> (105.8635, 10.5582)
  line L8 (105.8635, 10.5582) -> (97.8635, 10.5582)
  line L9 (105.8635, 10.5582) -> (97.8635, 10.5582) construction
  line L10 (105.8635, 14.8082) -> (97.8635, 14.8082)
  line L11 (97.8635, 6.3082) -> (105.8635, 6.3082)
  arc A18 (105.8635, 6.3082) -> (105.8635, 14.8082) centre (105.8635, 10.5582) ccw
  arc A19 (97.8635, 14.8082) -> (97.8635, 6.3082) centre (97.8635, 10.5582) ccw
  circle A20 centre (101.8635, 10.5582) radius 0.5
  dimension "d32" = 110
  dimension "d106" = 32
  dimension "d107" = 86.1011
  dimension "d108" = 110
  dimension "d109" = 55
  dimension "d119" = 5.6
  dimension "d120" = 5.6
  dimension "d121" = 55
  dimension "d122" = 80.54
  dimension "d123" = 25.36
  dimension "d124" = 8
  dimension "d125" = 8.5
  dimension "d126" = 1
  constraints: 18 end point, 9 point on circle, 8 centre point, 8 tangent, 3 coincident, 2 midpoint, 2 parallel, 2 point on line, 1 collinear, 1 concentric, 1 horizontal, 1 vertical alignment, 1 other
  measures "d106" diameter of A0
  measures "d107" diameter of A1
  measures "d108" distance of A1.centre A2.centre
  measures "d109" distance from line of A1.centre L1
  measures "d119" diameter of A14
  measures "d120" diameter of A5
  measures "d121" distance between parallel lines of L6 L1
  measures "d122" diameter of A17
  measures "d123" diameter of A16
  measures "d124" distance of L7.end L8.end
  measures "d125" diameter of A19
  measures "d126" diameter of A20
extrude "Extrusion8" cut sketch "Sketch13" against normal blind 6.35 contours A14 | A18 L11 A19 L10
sketch "Sketch14" plane through (0, 0, 6.35) normal (0, 0, 1) x (1, 0, 0)
  circle A0 centre (41.4015, -12.7853) radius 2.8 projected
  circle A1 centre (110.9985, -12.7853) radius 2.8 projected
  point P0 (0, 0)
extrude "Extrusion9" add sketch "Sketch14" against normal blind 6.35
fillet "Fillet3" radius 2 4 edges at (21.2, -92.5838, 3.175) (131.2, -92.5838, 3.175) (131.2, 117.4162, 3.175) (21.2, 117.4162, 3.175)
equation "\"d119\" = d120"
body "Solid1"
